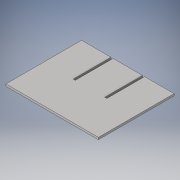
# Autodesk Inventor part: Wine Rack Horizontal
Saved by Autodesk Inventor 2016 (Build 200138000, 138)
## iProperties
Created: 2017-10-31
Part Number: Wine Rack Horizontal
Material: Generic
Document SubType Name: Modeling
Designer: mathaetaes
Density: 1 g/cm^3
Appearance: Default
Author: mathaetaes
Autodesk Inventor part; units mm, degrees
ref_plane "YZ Plane" through (0, 0, 0) normal (1, 0, 0) x (0, 1, 0)
ref_plane "XZ Plane" through (0, 0, 0) normal (0, 1, 0) x (-1, 0, 0)
ref_plane "XY Plane" through (0, 0, 0) normal (0, 0, 1) x (1, 0, 0)
sketch "Sketch1" plane through (0, 0, 0) normal (0, 1, 0) x (-1, 0, 0)
  line L0 (49.657, -96.9264) -> (-229.743, -96.9264)
  line L1 (-229.743, -96.9264) -> (-229.743, 131.6736)
  line L2 (-229.743, 131.6736) -> (49.657, 131.6736)
  line L3 (49.657, 131.6736) -> (49.657, -96.9264)
  point P0 (0, 0)
  dimension "d0" = 228.6
  dimension "d1" = 279.4
  constraints: 8 end point, 2 parallel, 1 horizontal, 1 perpendicular
  measures "d0" distance of L0.end L1.end
  measures "d1" distance of L0.start L0.end
extrude "Board" add sketch "Sketch1" along normal blind 6.35
sketch "Sketch2" plane through (0, 6.35, 0) normal (0, 1, 0) x (1, 0, 0)
  line L0 (39.243, 96.9264) -> (45.593, 96.9264)
  line L1 (45.593, 96.9264) -> (45.593, -17.3736)
  line L2 (45.593, -17.3736) -> (39.243, -17.3736)
  line L3 (39.243, -17.3736) -> (39.243, 96.9264)
  line L4 (-49.657, 96.9264) -> (-49.657, -131.6736) projected
  line L5 (134.493, 96.9264) -> (140.843, 96.9264)
  line L6 (140.843, 96.9264) -> (140.843, -17.3736)
  line L7 (140.843, -17.3736) -> (134.493, -17.3736)
  line L8 (134.493, -17.3736) -> (134.493, 96.9264)
  line L9 (229.743, -131.6736) -> (229.743, 96.9264) projected
  point P0 (0, 0)
  dimension "d4" = 6.35
  dimension "d5" = 114.3
  dimension "d6" = 88.9
  dimension "d7" = 6.35
  dimension "d8" = 114.3
  dimension "d13" = 88.9
  dimension "d17" = 88.9
  constraints: 16 end point, 4 parallel, 2 horizontal, 2 perpendicular
  measures "d4" distance of L0.start L0.end
  measures "d5" distance of L2.end L0.start
  measures "d6" distance between parallel lines of L4 L3
  measures "d7" distance of L5.start L5.end
  measures "d8" distance of L7.end L5.start
  measures "d13" distance between parallel lines of L8 L1
  measures "d17" distance between parallel lines of L9 L6
extrude "Extrusion2" cut sketch "Sketch2" against normal blind 6.35
equation "\"d5\" = 0.5 * d0"
equation "\"d8\" = 0.5 * d9"
equation "\"d9\" = 228.6"
body "Solid1"
